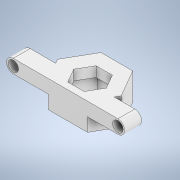
# Autodesk Inventor part: tensioner
Saved by Autodesk Inventor 2020 (Build 240168000, 168)
## iProperties
Created: 2021-03-17
Part Number: tensioner
Material: ABS Plastic
Document SubType Name: Modeling
Designer: AOB
Density: 1.06 g/cm^3
Appearance: Smooth - White
Mass: 1.43749 g
Surface Area: 14.094 cm^2
Volume: 1.35612 cm^3
Author: AOB
Autodesk Inventor part; units mm, degrees
ref_plane "YZ Plane" through (0, 0, 0) normal (1, 0, 0) x (0, 1, 0)
ref_plane "XZ Plane" through (0, 0, 0) normal (0, 1, 0) x (-1, 0, 0)
ref_plane "XY Plane" through (0, 0, 0) normal (0, 0, 1) x (1, 0, 0)
sketch "Sketch1" plane through (0, 0, 0) normal (0, 0, 1) x (1, 0, 0)
  line L0 (88.2444, -84.7287) -> (89.7444, -84.7287) construction
  circle A0 centre (12.0706, -84.7287) radius 1.55
  circle A1 centre (43.0706, -84.7287) radius 1.55
  arc A2 (12.0706, -82.7287) -> (12.0706, -86.7287) centre (12.0706, -84.7287) ccw
  arc A3 (43.0706, -86.7287) -> (43.0706, -82.7287) centre (43.0706, -84.7287) ccw
  line L1 (12.0706, -82.7287) -> (43.0706, -82.7287)
  line L2 (43.0706, -86.7287) -> (12.0706, -86.7287)
  point P0 (0, 0)
  dimension "d7" = 1.5
  dimension "d9" = 3.1
  dimension "d17" = 4
  dimension "d18" = 4
  dimension "d19" = 3.1
  constraints: 6 end point, 4 centre point, 4 point on circle, 3 tangent, 2 coincident, 1 horizontal
  measures "d7" distance of L0.start L0.end
  measures "d9" diameter of A1
  measures "d17" diameter of A2
  measures "d18" diameter of A3
  measures "d19" diameter of A0
extrude "Extrusion1" add sketch "Sketch1" along normal blind 5
sketch "Sketch2" plane through (12.0706, -82.7287, 0) normal (0, 1, 0) x (1, 0, 0)
  line L0 (0, 0) -> (31, 0) projected
  line L1 (0, -5) -> (31, -5) projected
  line L2 (15.5, -5) -> (15.5, -3.9958) construction
  line L3 (15.5, -3.9958) -> (10.5, -3.9958) construction
  line L4 (11.5085, 9.4605) -> (20.9225, 9.4605)
  line L5 (6.8015, 1.3078) -> (11.5085, 9.4605)
  line L6 (19.5, -4) -> (13.5, -4)
  line L7 (20.9225, 9.4605) -> (25.6295, 1.3078)
  line L8 (16.5, 6.3923) -> (16.5, 9.3923) construction
  line L9 (13.5, 6.3923) -> (19.5, 6.3923)
  line L10 (10.5, 1.1962) -> (13.5, 6.3923)
  line L11 (13.5, -4) -> (10.5, 1.1962)
  line L12 (19.5, -4) -> (13.5, -4)
  line L13 (22.5, 1.1962) -> (19.5, -4)
  line L14 (19.5, 6.3923) -> (22.5, 1.1962)
  line L15 (31, 0) -> (0, 0) projected
  line L16 (7.5565, 0) -> (24.8745, 0)
  line L17 (6.8015, 1.3078) -> (7.5565, 0)
  line L18 (25.6295, 1.3078) -> (21.9877, -5)
  line L19 (7.5565, 0) -> (10.4433, -5)
  line L20 (10.4433, -5) -> (21.9877, -5)
  line L21 (31, -5) -> (0, -5) projected
  point P0 (-12.0706, 0)
  point P1 (12, 3.6023)
  point P2 (12, -1.5939)
  point P3 (16.5, -4.192)
  point P4 (21, -1.5939)
  point P5 (20.9225, 9.4605)
  point P6 (25.6295, 1.3078)
  point P7 (21, 3.6023)
  point P8 (11.1906, 0)
  point P9 (13.5, -4)
  point P10 (21.8094, 0)
  point P11 (10.5, 1.1962)
  point P12 (11.1906, 0)
  point P13 (21.8094, 0)
  point P14 (25.6295, 1.3078)
  dimension "d23" = 5
  dimension "d44" = 3
  constraints: 30 end point, 3 point on line, 2 vertical, 1 collinear, 1 horizontal, 1 midpoint, 9 other
  measures "d23" distance of L2.end L3.end
  measures "d44" distance of L8.start L8.end
extrude "Extrusion2" cut sketch "Sketch2" against normal through all contours L0 L13 L6 L11
sketch "Sketch6" plane through (12.0706, -82.7287, 5) normal (0, 1, 0) x (1, 0, 0)
  line L0 (14.179, 10.3462) -> (11.761, 6.1581)
  line L1 (11.761, 6.1581) -> (14.179, 1.97)
  line L2 (19.015, 1.97) -> (21.433, 6.1581)
  line L3 (19.015, 10.3462) -> (21.433, 6.1581)
  line L4 (14.179, 10.3462) -> (19.015, 10.3462)
  line L5 (14.179, 1.97) -> (19.015, 1.97)
  line L6 (10.5, 6.1962) -> (13.5, 11.3923) projected
  line L7 (13.5, 11.3923) -> (19.5, 11.3923) projected
  line L8 (19.5, 11.3923) -> (22.5, 6.1962) projected
  line L9 (13.5, 1) -> (10.5, 6.1962) projected
  line L10 (19.5, 1) -> (13.5, 1) projected
  line L11 (21.8094, 5) -> (19.5, 1) projected
  line L12 (22.5, 6.1962) -> (19.5, 1) projected
  constraints: 12 end point, 2 parallel
extrude "Extrusion11" add sketch "Sketch2" against normal blind 8 contours L17 L5 L4 L7 L18 L0 L13 L14 L9 L10 L11 | L0 L11 L6 L13 L18 L1 L19
extrude "Extrusion12" add sketch "Sketch6" against normal blind 3
body "Solid3"
